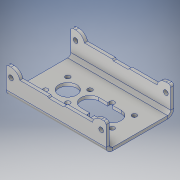
# Autodesk Inventor part: Servo_Bracket
Saved by Autodesk Inventor 2019 (Build 230136000, 136)
## iProperties
Created: 2021-02-23
Part Number: Servo_Bracket
Material: Aluminum 6061
Document SubType Name: Sheet Metal
Designer: zhanb
Density: 2.7 g/cm^3
Sheet Metal Rule: Default
Appearance: Aluminum - Flat
Author: zhanb
Autodesk Inventor part; units mm, degrees
ref_plane "YZ Plane" through (0, 0, 0) normal (1, 0, 0) x (0, 1, 0)
ref_plane "XZ Plane" through (0, 0, 0) normal (0, 1, 0) x (-1, 0, 0)
ref_plane "XY Plane" through (0, 0, 0) normal (0, 0, 1) x (1, 0, 0)
sketch "Sketch1" plane through (0, 0, 0) normal (0, 1, 0) x (-1, 0, 0)
  line L0 (-22.25, 12.295) -> (22.25, 12.295)
  line L1 (22.25, 12.295) -> (22.25, -12.295)
  line L2 (22.25, -12.295) -> (-22.25, -12.295)
  line L3 (-22.25, -12.295) -> (-22.25, 12.295)
  line L4 (-22.25, 12.295) -> (22.25, -12.295) construction
  line L5 (22.25, 12.295) -> (-22.25, -12.295) construction
  point P0 (0, 0)
  dimension "d0" = 24.59
  dimension "d1" = 44.5
  measures "d0" distance of L0.end L1.end
  measures "d1" distance of L0.start L0.end
extrude "Plate1" add sketch "Sketch1" along normal blind 1.4
sketch "Sketch2" plane through (0, 1.4, 0) normal (0, 1, 0) x (1, 0, 0)
  line L0 (-14.8492, -4.9497) -> (-4.9497, -4.9497) construction
  line L1 (-4.9497, -4.9497) -> (-4.9497, 4.9497) construction
  line L2 (-4.9497, 4.9497) -> (-14.8492, 4.9497) construction
  line L3 (-14.8492, 4.9497) -> (-14.8492, -4.9497) construction
  line L4 (-14.8492, -4.9497) -> (-4.9497, 4.9497) construction
  line L5 (-4.9497, -4.9497) -> (-14.8492, 4.9497) construction
  line L6 (-4.9497, -4.9497) -> (4.9497, -4.9497) construction
  line L7 (4.9497, -4.9497) -> (4.9497, 4.9497) construction
  line L8 (4.9497, 4.9497) -> (-4.9497, 4.9497) construction
  line L9 (-4.9497, 4.9497) -> (-4.9497, -4.9497) construction
  line L10 (4.9497, -4.9497) -> (14.8492, -4.9497) construction
  line L11 (14.8492, -4.9497) -> (14.8492, 4.9497) construction
  line L12 (14.8492, 4.9497) -> (4.9497, 4.9497) construction
  line L13 (4.9497, 4.9497) -> (4.9497, -4.9497) construction
  line L14 (-4.9497, -4.9497) -> (4.9497, 4.9497) construction
  circle A0 centre (-9.8995, 0) radius 4
  line L15 (0, -4) -> (9.8995, -4)
  line L16 (9.8995, 4) -> (0, 4)
  arc A1 (0, 4) -> (0, -4) centre (0, 0) ccw
  arc A2 (9.8995, -4) -> (9.8995, 4) centre (9.8995, 0) ccw
  arc A3 (5.9997, -4.9497) -> (3.8997, -4.9497) centre (4.9497, -4.9497) ccw construction
  arc A4 (3.8997, 4.9497) -> (5.9997, 4.9497) centre (4.9497, 4.9497) ccw construction
  line L17 (3.8997, -4.9497) -> (3.8997, 4.9497)
  line L18 (5.9997, 4.9497) -> (5.9997, -4.9497)
  arc A5 (3.8997, -4.9497) -> (5.9997, -4.9497) centre (4.9497, -4.9497) ccw
  arc A6 (5.9997, 4.9497) -> (3.8997, 4.9497) centre (4.9497, 4.9497) ccw
  point P0 (9.8995, -4.9497)
  dimension "d3" = 14
  dimension "d4" = 8
  dimension "d14" = 1.05
  constraints: 38 end point, 13 coincident, 12 point on circle, 7 centre point, 7 parallel, 6 perpendicular, 5 point on line, 4 horizontal, 4 midpoint, 3 equal radius, 3 tangent, 1 vertical alignment
  measures "d3" distance of L1.end L0.start
  measures "d4" diameter of A0
  measures "d14" radius of A5
hole "Hole1" at (-14.8492, 1.4, 4.9497) at (-4.9497, 1.4, 4.9497) at (4.9497, 1.4, 4.9497) at (14.8492, 1.4, 4.9497) at (14.8492, 1.4, -4.9497) at (4.9497, 1.4, -4.9497) at (-4.9497, 1.4, -4.9497) at (-14.8492, 1.4, -4.9497) direction (0, -1, 0) diameter 2.1 end through all both
extrude "Cut1" cut sketch "Sketch2" against normal blind 1.4
sketch "Sketch3" plane through (22.25, 2.8, 13.695) normal (0, 0, 1) x (1, 0, 0)
  line L0 (-44.5, 0) -> (0, 0)
  line L1 (0, 0) -> (0, 9.77)
  line L2 (0, 9.77) -> (-44.5, 9.77)
  line L3 (-44.5, 9.77) -> (-44.5, 0)
  constraints: 6 end point, 1 horizontal, 1 perpendicular, 1 vertical
edge flange "Flange1" height 12.57 angle 90 thickness 1.4 bend radius 1.4 thickness toward (0, 0, 1) relief straight relief width 1.4 relief depth 0.7 corner gap 1.4 corner form 0 edges at (0, 1.4, 12.295) (0, 1.4, -12.295) wall of the first edge with corners at (-22.25, 2.8, 13.695) (22.25, 2.8, 13.695) (22.25, 12.57, 13.695) (-22.25, 12.57, 13.695)
bend "Bend1"
corner "Corner1"
sketch "Sketch4" plane through (-22.25, 12.57, 15.095) normal (0, 0, 1) x (1, 0, 0)
  line L0 (0, -9.77) -> (44.5, -9.77) construction
  line L1 (44.5, 0) -> (44.5, -9.77) construction
  line L2 (0, 0) -> (44.5, 0) construction
  line L3 (0, -9.77) -> (0, 0) construction
  line L4 (2.15, -4.07) -> (42.35, -4.07) construction
  line L5 (44.5, -12.57) -> (0, -12.57) projected
  line L6 (44.5, 0) -> (0, 0) projected
  arc A0 (42.35, 0) -> (38.4048, -3.07) centre (42.35, -4.07) ccw
  arc A1 (6.0952, -3.07) -> (2.15, 0) centre (2.15, -4.07) ccw
  line L7 (6.0952, -3.07) -> (18.5, -3.07)
  line L8 (18.5, -3.07) -> (19, -3.57)
  line L9 (19, -3.57) -> (25.5, -3.57)
  line L10 (25.5, -3.57) -> (26, -3.07)
  line L11 (26, -3.07) -> (38.4048, -3.07)
  line L12 (22.25, -4.07) -> (22.25, 0) construction
  line L13 (44.5, -9.77) -> (44.5, 0) projected
  arc A2 (44.5, -1) -> (43.5, 0) centre (43.5, -1) ccw
  line L14 (0, 0) -> (0, -9.77) projected
  arc A3 (1, 0) -> (0, -1) centre (1, -1) ccw
  line L15 (44.5, 0) -> (44.5, -9.77) projected
  line L16 (0, 0) -> (44.5, 0) projected
  line L17 (0, -1) -> (0, 1)
  line L18 (0, 1) -> (44.5, 1)
  line L19 (44.5, 1) -> (44.5, -1)
  line L20 (42.35, 0) -> (43.5, 0)
  line L21 (1, 0) -> (2.15, 0)
  dimension "d26" = 8.5
  dimension "d27" = 40.2
  dimension "d35" = 0.5
  dimension "d36" = 1
  dimension "d37" = 6.5
  dimension "d38" = 135
  dimension "d39" = 1
  dimension "d40" = 1
  constraints: 24 end point, 8 point on circle, 8 point on line, 4 centre point, 4 tangent, 3 collinear, 3 horizontal, 2 coincident, 2 midpoint, 1 equal radius, 1 parallel, 1 perpendicular, 1 vertical, 1 vertical alignment, 4 other
  measures "d26" distance between parallel lines of L5 L4
  measures "d27" distance of L4.start L4.end
  measures "d35" distance between parallel lines of L7 L9
  measures "d36" distance between parallel lines of L4 L7
  measures "d37" distance of L8.end L9.end
  measures "d38" angle of L7 L8
  measures "d39" radius of A2
  measures "d40" distance between parallel lines of L2 L18
hole "Hole2" at (-20.1, 8.5, 15.095) at (20.1, 8.5, 15.095) direction (0, 0, -1) diameter 2.1 end through all both
extrude "Cut2" cut sketch "Sketch4" along normal through all both and the other way through all contours L13 A2 L6 | A0 L11 L10 L9 L8 L7 A1 L6 | L6 A3 L14
equation "\"d10\" = Thickness"
equation "\"d12\" = Thickness"
equation "\"d33\" = Thickness"
equation "\"d41\" = Thickness"
equation "\"d2\" = Thickness"
equation "\"d15\" = BendReliefWidth"
equation "\"d16\" = BendReliefDepth"
equation "\"d17\" = MinimumRemnant"
equation "\"d18\" = TransitionRadius"
equation "\"d21\" = BendRadius"
equation "\"d22\" = CornerReliefSize"
equation "\"d23\" = GapSize"
equation "\"d24\" = JacobiRadiusSize"
equation "\"BendRadius\" = Thickness"
equation "\"BendReliefWidth\" = Thickness"
equation "\"BendReliefDepth\" = 0.5 * Thickness"
equation "\"CornerReliefSize\" = 4 * Thickness"
equation "\"MinimumRemnant\" = 2 * Thickness"
equation "\"TransitionRadius\" = BendRadius"
equation "\"JacobiRadiusSize\" = Thickness"
equation "\"GapSize\" = Thickness"
equation "\"Thickness\" = 1.4"
body "Solid1"
